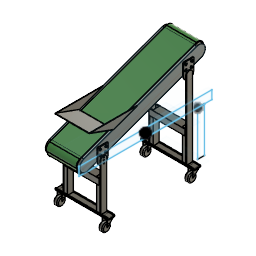
Conveyor Belt with Hopper (Autodesk Fusion 360 design; units mm, degrees)
Autodesk Fusion 360 part; units mm, degrees
note: some values were not read from the file. Chosen so that the rebuilt part matches the saved one: which bodies a step acts on; which face or edge a step refers to. Set by a fixed rule: which sketch regions a step uses.
sketch "Sketch1" plane through (0, 0, 0) normal (1, 0, 0) x (0, 1, 0)
  line L0 (775, 50) -> (-775, 50)
  line L1 (-775, 50) -> (-775, -50)
  line L2 (-775, -50) -> (775, -50)
  line L3 (775, -50) -> (775, 50)
  dimension "d1" = 1550
  dimension "d2" = 100
  constraint horizontal L0
  constraint perpendicular L0 L1
  constraint parallel L0 L2
  constraint parallel L1 L3
  measures "d1" distance of L1.end L2.end
  measures "d2" distance of L0.end L1.end
extrude "Extrude1" add sketch "Sketch1" against normal blind 400 makes body 1
extrude "Extrude2" add 1 faces at (-133.3333, 258.3333, 50) along direction (0, 0, 1) blind 100 on bodies 1 bodies 1
extrude "Extrude3" cut 1 faces at (-133.3333, 258.3333, 150) along direction (0, 0, -1) blind 50 on bodies 1 bodies 1
fillet "Fillet1" radius 75 4 edges at (-200, -775, 100) (-200, -775, -50) (-200, 775, 100) (-200, 775, -50) on bodies 1
sketch "Sketch2" plane through (0, 0, 0) normal (0, 1, 0) x (1, 0, 0)
sketch "Sketch3" plane through (0, 0, 0) normal (1, 0, 0) x (0, 1, 0)
  arc A0 (700, -50) -> (700, 100) centre (700, 25) ccw
  line L0 (700, 100) -> (-700, 100)
  arc A1 (-700, 100) -> (-700, -50) centre (-700, 25) ccw
  line L1 (-700, -50) -> (700, -50)
  line L2 (608.0223, -50) -> (688.0223, -50)
  line L3 (688.0223, -50) -> (688.0223, -570)
  line L4 (688.0223, -570) -> (608.0223, -570)
  line L5 (608.0223, -570) -> (608.0223, -50)
  dimension "d11" = 80
  dimension "d12" = 520
  constraint horizontal L2
  constraint vertical L3
  constraint horizontal L4
  constraint vertical L5
  constraint coincident L1 L2.start
  measures "d11" distance of L2.start L2.end
  measures "d12" distance of L2.start L4.end
sketch "Sketch4" plane through (0, 0, 0) normal (1, 0, 0) x (0, 1, 0)
  arc A0 (700, -50) -> (700, 100) centre (700, 25) ccw
  line L0 (700, 100) -> (-700, 100)
  arc A1 (-700, 100) -> (-700, -50) centre (-700, 25) ccw
  line L1 (-700, -50) -> (700, -50)
  line L2 (655, 125) -> (555, 125)
  line L3 (555, 125) -> (555, -75)
  line L4 (555, -75) -> (655, -75)
  line L5 (655, -75) -> (655, 125)
  point P0 (605, 25)
  dimension "d16" = 100
  dimension "d17" = 200
  constraint horizontal L2
  constraint perpendicular L2 L3
  constraint parallel L2 L4
  constraint parallel L3 L5
  measures "d16" distance of L3.end L4.end
  measures "d17" distance of L2.end L3.end
extrude "Extrude5" add sketch "Sketch4" along normal blind 10 separate body contours L1 L3 L4 L5 | L0 L1 L3 L5 | L0 L2 L3 L5 makes body 2
move_body "Move1" bodies 2 to x (1, 0, 0) y (0, 1, 0) z (0, 0, 1) at (0, 0, -50)
extrude "Extrude6" add 3 faces at (3.3333, 555, 66.6667) (6.6667, 555, 0) (3.3333, 555, -108.3333) along direction (0, -1, 0) blind 20 on bodies 2 bodies 1 2
sketch "Sketch5" plane through (10, 0, 0) normal (1, 0, 0) x (0, 1, 0)
  line L0 (655, -125) -> (655, 75)
  line L1 (655, 75) -> (535, 75)
  line L2 (535, 75) -> (535, -125)
  line L3 (535, -125) -> (655, -125)
  line L4 (595, 75) -> (595, -45)
  line L5 (620, 215) -> (570, 215)
  line L6 (570, 215) -> (570, -305)
  line L7 (570, -305) -> (620, -305)
  line L8 (620, -305) -> (620, 215)
  point P0 (595, -45)
  dimension "d22" = 120
  dimension "d23" = 50
  dimension "d24" = 520
  constraint midpoint L1 L4.start
  constraint perpendicular L1 L4
  constraint horizontal L5
  constraint perpendicular L5 L6
  constraint parallel L5 L7
  constraint parallel L6 L8
  constraint coincident P0 L4.end
  measures "d22" distance of L4.start P0
  measures "d23" distance of L6.end L7.end
  measures "d24" distance of L5.end L6.end
extrude "Extrude7" add sketch "Sketch5" along normal blind 10 separate body contours L3 L6 L7 L8 | L1 L3 L6 L8 | L1 L5 L6 L8 makes body 3
move_body "Move2" bodies 3 to x (1, 0, 0) y (0, 1, 0) z (0, 0, 1) at (0, 0, -260)
move_body "Move3" bodies 3 to x (1, 0, 0) y (0, 1, 0) z (0, 0, 1) at (0, 0, 20)
extrude "Extrude8" add 3 faces at (16.6667, 620, -485) (16.6667, 620, -298.3333) (16.6667, 620, -118.3333) along direction (0, 1, 0) blind 20 on bodies 3 bodies 3
move_body "Move4" bodies 3 to x (1, 0, 0) y (0, 1, 0) z (0, 0, 1) at (0, -10, 0)
fillet "Fillet2" radius 35 2 edges at (15, 630, -25) (15, 560, -25) on bodies 3
fillet "Fillet3" radius 60 2 edges at (5, 535, -125) (5, 655, -125) on bodies 1
sketch "Sketch6" plane through (10, 0, 0) normal (-1, 0, 0) x (0, -1, 0)
  arc A0 (-560, -60) -> (-630, -60) centre (-595, -60) ccw
  line L0 (-630, -60) -> (-630, -545)
  line L1 (-630, -545) -> (-560, -545)
  line L2 (-560, -545) -> (-560, -60)
sketch "Sketch7" plane through (20, 0, 0) normal (1, 0, 0) x (0, 1, 0)
  arc A0 (630, -60) -> (560, -60) centre (595, -60) ccw
  line L0 (560, -60) -> (560, -545)
  line L1 (560, -545) -> (630, -545)
  line L2 (630, -545) -> (630, -60)
  line L3 (595, -25) -> (595, -225)
  line L4 (630, -545) -> (560, -545)
  line L5 (560, -545) -> (560, -225)
  line L6 (560, -225) -> (630, -225)
  line L7 (630, -225) -> (630, -545)
  dimension "d33" = 200
  constraint midpoint A0 L3.start
  constraint vertical L3
  constraint horizontal L4
  constraint vertical L5
  constraint horizontal L6
  constraint vertical L7
  constraint coincident L0 L5.end
  constraint coincident L1.end L2.start
  measures "d33" distance of L3.start L3.end
extrude "Extrude9" add sketch "Sketch7" along normal blind 20 separate body contours L0 L1 L2 L4 L5 L6 L7 makes body 4
move_body "Move5" bodies 4 to x (1, 0, 0) y (0, 1, 0) z (0, 0, 1) at (-30, 0, 0)
extrude "Extrude10" add 1 faces at (-10, 595, -438.3333) along direction (-1, 0, 0) blind 20 on bodies 4 bodies 4
sketch "Sketch8" plane through (0, 0, 0) normal (0, 1, 0) x (1, 0, 0)
sketch "Sketch9" plane through (0, 0, 0) normal (0, 1, 0) x (1, 0, 0)
  line L0 (-50, 190) -> (-450, 190)
  line L1 (-450, 190) -> (-450, 240)
  line L2 (-450, 240) -> (-50, 240)
  line L3 (-50, 240) -> (-50, 190)
  dimension "d38" = 400
  dimension "d39" = 50
  constraint horizontal L0
  constraint vertical L1
  constraint horizontal L2
  constraint vertical L3
  measures "d38" distance of L0.start L0.end
  measures "d39" distance of L0.start L2.end
extrude "Extrude11" add sketch "Sketch9" along normal blind 90 separate body makes body 5
move_body "Move6" bodies 5 to x (1, 0, 0) y (0, 1, 0) z (0, 0, 1) at (50, 550, 30)
extrude "Extrude12" add 1 faces at (-133.3333, 580, -160) along direction (0, 0, 1) blind 20 on bodies 5 bodies 5
sketch "Sketch10" plane through (0, 0, -210) normal (0, 0, -1) x (1, 0, 0)
  line L0 (0, -550) -> (-400, -550)
  line L1 (-400, -550) -> (-400, -640)
  line L2 (-400, -640) -> (0, -640)
  line L3 (0, -640) -> (0, -550)
sketch "Sketch11" plane through (0, 0, -210) normal (0, 0, -1) x (1, 0, 0)
  line L0 (0, -630) -> (-40, -630)
  line L1 (-40, -630) -> (-40, -560)
  line L2 (-40, -560) -> (0, -560)
  line L3 (0, -560) -> (0, -630)
  dimension "d44" = 40
  dimension "d45" = 70
  constraint horizontal L0
  constraint vertical L1
  constraint horizontal L2
  constraint vertical L3
  measures "d44" distance of L0.start L0.end
  measures "d45" distance of L0.start L2.end
sketch "Sketch12" plane through (0, 0, -210) normal (0, 0, -1) x (1, 0, 0)
  line L0 (-400, -630) -> (-360, -630)
  line L1 (-360, -630) -> (-360, -560)
  line L2 (-360, -560) -> (-400, -560)
  line L3 (-400, -560) -> (-400, -630)
  dimension "d46" = 40
  dimension "d47" = 70
  constraint horizontal L0
  constraint vertical L1
  constraint horizontal L2
  constraint vertical L3
  measures "d46" distance of L0.start L0.end
  measures "d47" distance of L0.start L2.end
extrude "Extrude13" cut sketch "Sketch11" sketch "Sketch12" against normal blind 75 of sketch 2 bodies 5
move_body "Move7" bodies 5 to x (1, 0, 0) y (0, 1, 0) z (0, 0, 1) at (10, 0, -40)
sketch "Sketch13" plane through (0, 0, -50) normal (0, 0, -1) x (1, 0, 0)
  line L0 (-400, -700) -> (0, -700)
  line L1 (0, -700) -> (0, -655)
  line L2 (0, -655) -> (0, -535)
  line L3 (0, -535) -> (0, 700)
  line L4 (0, 700) -> (-400, 700)
  line L5 (-400, 700) -> (-400, -700)
sketch "Sketch14" plane through (0, 0, -545) normal (0, 0, -1) x (1, 0, 0)
  line L0 (-30, -630) -> (10, -630)
  line L1 (10, -630) -> (10, -560)
  line L2 (10, -560) -> (-30, -560)
  line L3 (-30, -560) -> (-30, -630)
  line L4 (10, -560) -> (-390, -560)
  line L5 (-390, -560) -> (-390, -610)
  line L6 (-390, -610) -> (10, -610)
  line L7 (10, -610) -> (10, -560)
  dimension "d50" = 400
  dimension "d51" = 50
  constraint horizontal L4
  constraint vertical L5
  constraint horizontal L6
  constraint vertical L7
  constraint coincident L1.end L2.start
  measures "d50" distance of L1.end L4.end
  measures "d51" distance of L1.end L6.end
extrude "Extrude14" add sketch "Sketch14" along normal blind 10 separate body contours L3 L4 L5 L6 | L1 L2 L3 L4 L6 L7 makes body 6
extrude "Extrude15" add 1 faces at (10, 593.3333, -548.3333) along direction (1, 0, 0) blind 100 on bodies 6 bodies 6
extrude "Extrude16" add 1 faces at (-223.3333, 610, -548.3333) along direction (0, 1, 0) blind 20 on bodies 6 bodies 6
extrude "Extrude17" add 1 faces at (-223.3333, 630, -548.3333) along direction (0, 1, 0) blind 5 on bodies 6 bodies 6
sketch "Sketch15" plane through (0, 0, -545) normal (0, 0, 1) x (-1, 0, 0)
  line L0 (390, -635) -> (390, -560)
  line L1 (390, -560) -> (-110, -560)
  line L2 (-110, -560) -> (-110, -635)
  line L3 (-110, -635) -> (390, -635)
sketch "Sketch16" plane through (0, 0, -545) normal (0, 0, 1) x (-1, 0, 0)
  line L0 (-110, -560) -> (390, -560)
  line L1 (390, -560) -> (390, -565)
  line L2 (390, -565) -> (-110, -565)
  line L3 (-110, -565) -> (-110, -560)
  line L4 (-110, -635) -> (390, -635)
  line L5 (390, -635) -> (390, -630)
  line L6 (390, -630) -> (-110, -630)
  line L7 (-110, -630) -> (-110, -635)
  dimension "d60" = 500
  dimension "d61" = 5
  dimension "d62" = 500
  dimension "d63" = 5
  constraint horizontal L0
  constraint vertical L1
  constraint horizontal L2
  constraint vertical L3
  constraint horizontal L4
  constraint vertical L5
  constraint horizontal L6
  constraint vertical L7
  measures "d60" distance of L0.start L0.end
  measures "d61" distance of L0.start L2.end
  measures "d62" distance of L4.start L4.end
  measures "d63" distance of L4.start L6.end
extrude "Extrude18" add sketch "Sketch16" along normal blind 10 bodies 6
sketch "Sketch17" plane through (20, 0, 0) normal (1, 0, 0) x (0, 1, 0)
  arc A0 (630, -60) -> (560, -60) centre (595, -60) ccw
  line L0 (560, -60) -> (560, -545)
  line L1 (560, -545) -> (630, -545)
  line L2 (630, -545) -> (630, -60)
  circle A1 centre (600, -675) radius 50
  dimension "d66" = 100
  measures "d66" diameter of A1
extrude "Extrude19" add sketch "Sketch17" along normal blind 50 separate body contours A1 makes body 7
sketch "Sketch18" plane through (70, 0, 0) normal (1, 0, 0) x (0, 1, 0)
  circle A0 centre (600, -675) radius 50
  line L0 (675, -600) -> (600, -600)
  line L1 (600, -600) -> (600, -675)
  line L2 (600, -675) -> (675, -600)
  dimension "d70" = 75
  constraint horizontal L0
  constraint vertical L1
  constraint coincident A0.centre L1.end
  measures "d70" distance of A0.centre L0.end
extrude "Extrude20" add sketch "Sketch18" along normal blind 5 separate body contours A0 L1 L2 | A0 L0 L1 L2 picked at (618.4794, -647.3437) makes body 8
extrude "Extrude21" add 1 faces at (73.3333, 650, -600) along direction (0, 0, 1) blind 10 on bodies 8 bodies 8
copy_body "CopyPasteBodies1" bodies 8 makes body 9
move_body "Move8" bodies 9 to x (1, 0, 0) y (0, 1, 0) z (0, 0, 1) at (-55, 0, 0)
move_body "Move9" bodies 7 8 9 to x (1, 0, 0) y (0, 1, 0) z (0, 0, 1) at (20, -40, 35)
sketch "Sketch19" plane through (0, 0, 0) normal (1, 0, 0) x (0, 1, 0)
sketch "Sketch20" plane through (0, 0, 0) normal (1, 0, 0) x (0, 1, 0)
  line L0 (-50, 100) -> (-1500, 100)
  line L1 (-1550, 50) -> (-1550, 0)
  line L2 (-1500, -50) -> (-75, -50)
  line L3 (0, 25) -> (0, 50)
  arc A0 (-1550, 0) -> (-1500, -50) centre (-1500, 0) ccw
  arc A1 (-1500, 100) -> (-1550, 50) centre (-1500, 50) ccw
  arc A2 (0, 50) -> (-50, 100) centre (-50, 50) ccw
  arc A3 (-75, -50) -> (0, 25) centre (-75, 25) ccw
  line L4 (-1560, 50) -> (-1560, 0)
  arc A4 (-1560, 0) -> (-1500, -60) centre (-1500, 0) ccw
  line L5 (-1500, -60) -> (-75, -60)
  arc A5 (-75, -60) -> (10, 25) centre (-75, 25) ccw
  line L6 (10, 25) -> (10, 50)
  arc A6 (10, 50) -> (-50, 110) centre (-50, 50) ccw
  line L7 (-50, 110) -> (-1500, 110)
  arc A7 (-1500, 110) -> (-1560, 50) centre (-1500, 50) ccw
  point P0 (-1550, 100)
  point P1 (-1550, -50)
  point P2 (0, -50)
  point P3 (-775, 25)
  dimension "d75" = 1550
  dimension "d76" = 150
  dimension "d77" = 50
  dimension "d78" = 75
  dimension "d79" = 10
  constraint horizontal L0
  constraint perpendicular L0 L1
  constraint parallel L0 L2
  constraint parallel L1 L3
  constraint coincident P1 L2
  constraint coincident P1 L1
  constraint tangent L2 A0
  constraint tangent L1 A0
  constraint coincident P0 L0
  constraint coincident P0 L1
  constraint tangent L0 A1
  constraint tangent L1 A1
  constraint equal A0 A1
  constraint tangent L3 A2
  constraint tangent L0 A2
  constraint equal A0 A2
  constraint coincident P2 L2
  constraint coincident P2 L3
  constraint tangent L2 A3
  constraint tangent L3 A3
  measures "d75" distance of P1 P2
  measures "d76" distance of P0 P1
  measures "d77" radius of A0
  measures "d78" radius of A3
extrude "Extrude22" add sketch "Sketch20" along normal blind 350 separate body makes body 10
move_body "Move10" bodies 10 to x (1, 0, 0) y (0, 1, 0) z (0, 0, 1) at (-375, 780, 0)
sketch "Sketch21" plane through (10, 0, 0) normal (1, 0, 0) x (0, 1, 0)
  arc A0 (535, -65) -> (655, -65) centre (595, -65) ccw
  line L0 (655, -65) -> (655, 75)
  line L1 (655, 75) -> (535, 75)
  line L2 (535, 75) -> (535, -65)
  circle A1 centre (580, 180) radius 12.5
  dimension "d83" = 25
  measures "d83" diameter of A1
extrude "Extrude23" add sketch "Sketch21" along normal blind 5 separate body contours A1 makes body 11
move_body "Move11" bodies 11 to x (1, 0, 0) y (0, 1, 0) z (0, 0, 1) at (0, -20, -130)
move_body "Move12" bodies 11 to x (1, 0, 0) y (0, 1, 0) z (0, 0, 1) at (0, 0, 150)
sketch "Sketch22" plane through (15, 0, 0) normal (1, 0, 0) x (0, 1, 0)
  circle A0 centre (560, 200) radius 12.5
  line L0 (555.3812, 208) -> (550.7624, 200)
  line L1 (550.7624, 200) -> (555.3812, 192)
  line L2 (555.3812, 192) -> (564.6188, 192)
  line L3 (564.6188, 192) -> (569.2376, 200)
  line L4 (569.2376, 200) -> (564.6188, 208)
  line L5 (564.6188, 208) -> (555.3812, 208)
  point P0 (560, 200)
  dimension "d86" = 8
  constraint coincident P0 A0.centre
  measures "d86" distance of P0 L5
extrude "Extrude24" cut sketch "Sketch22" against normal blind 4 contours L0 L1 L2 L3 L4 L5 bodies 11
move_body "Move13" bodies 11 to x (1, 0, 0) y (0, 1, 0) z (0, 0, 1) at (0, 0, -150)
copy_body "CopyPasteBodies2" bodies 11 makes body 12
move_body "Move14" bodies 12 to x (1, 0, 0) y (0, 1, 0) z (0, 0, 1) at (0, 65, 0)
copy_body "CopyPasteBodies3" bodies 11 12 makes body 13 makes body 14
move_body "Move15" bodies 13 14 to x (1, 0, 0) y (0, 1, 0) z (0, 0, 1) at (0, 0, -60)
move_body "Move16" bodies 12 to x (1, 0, 0) y (0, 1, 0) z (0, 0, 1) at (0, 4, 0)
sketch "Sketch23" plane through (10, 0, 0) normal (-1, 0, 0) x (0, -1, 0)
sketch "Sketch24" plane through (20, 0, 0) normal (1, 0, 0) x (0, 1, 0)
  arc A0 (630, -60) -> (560, -60) centre (595, -60) ccw
  line L0 (560, -60) -> (560, -545)
  line L1 (560, -545) -> (630, -545)
  line L2 (630, -545) -> (630, -60)
  circle A1 centre (480, -120) radius 5
  dimension "d89" = 10
  measures "d89" diameter of A1
extrude "Extrude25" add sketch "Sketch24" along normal blind 5 separate body contours A1 makes body 15
sketch "Sketch25" plane through (25, 0, 0) normal (1, 0, 0) x (0, 1, 0)
  circle A0 centre (480, -120) radius 5
  line L0 (477.9793, -116.5) -> (475.9585, -120)
  line L1 (475.9585, -120) -> (477.9793, -123.5)
  line L2 (477.9793, -123.5) -> (482.0207, -123.5)
  line L3 (482.0207, -123.5) -> (484.0415, -120)
  line L4 (484.0415, -120) -> (482.0207, -116.5)
  line L5 (482.0207, -116.5) -> (477.9793, -116.5)
  point P0 (480, -120)
  dimension "d92" = 3.5
  constraint coincident P0 A0.centre
  measures "d92" distance of P0 L5
extrude "Extrude26" cut sketch "Sketch25" against normal blind 4 contours L0 L1 L2 L3 L4 L5 bodies 15
move_body "Move17" bodies 15 to x (1, 0, 0) y (0, 1, 0) z (0, 0, 1) at (0, 115, 80)
move_body "Move18" bodies 15 to x (1, 0, 0) y (0, 1, 0) z (0, 0, 1) at (0, -2, 0)
copy_body "CopyPasteBodies4" bodies 15 makes body 16
move_body "Move19" bodies 16 to x (1, 0, 0) y (0, 1, 0) z (0, 0, 1) at (0, 0, -20)
copy_body "CopyPasteBodies5" bodies 15 makes body 17
move_body "Move20" bodies 17 to x (1, 0, 0) y (0, 1, 0) z (0, 0, 1) at (0, 0, -40)
move_body "Move21" bodies 16 to x (1, 0, 0) y (0, 1, 0) z (0, 0, 1) at (0, 0, -10)
move_body "Move22" bodies 17 to x (1, 0, 0) y (0, 1, 0) z (0, 0, 1) at (0, 0, -20)
sketch "Sketch26" plane through (20, 0, 0) normal (1, 0, 0) x (0, 1, 0)
  arc A0 (630, -60) -> (560, -60) centre (595, -60) ccw
  line L0 (560, -60) -> (560, -545)
  line L1 (560, -545) -> (630, -545)
  line L2 (630, -545) -> (630, -60)
  line L3 (742.0156, -320.3349) -> (703.7134, -288.1956)
  line L4 (697.2855, -295.856) -> (735.5877, -327.9954)
  arc A1 (703.7134, -288.1956) -> (696.6692, -288.8119) centre (700.4994, -292.0258) ccw
  arc A2 (696.6692, -288.8119) -> (697.2855, -295.856) centre (700.4994, -292.0258) ccw
  arc A3 (742.6319, -327.3791) -> (742.0156, -320.3349) centre (738.8017, -324.1652) ccw
  arc A4 (735.5877, -327.9954) -> (742.6319, -327.3791) centre (738.8017, -324.1652) ccw
  point P0 (692.2227, -278.5538)
  point P1 (685.7948, -286.2142)
  point P2 (731.7575, -324.7815)
  point P3 (727.2189, -297.3016)
  dimension "d95" = 60
  dimension "d96" = 10
  dimension "d97" = 5
  constraint parallel L3 L4
  constraint coincident P0 L3
  constraint tangent L3 A1
  constraint coincident P1 L4
  constraint tangent L4 A2
  constraint equal A1 A2
  constraint coincident A1.end A2.start
  constraint tangent L3 A3
  constraint equal A1 A3
  constraint coincident P2 L4
  constraint tangent L4 A4
  constraint equal A1 A4
  constraint coincident A3.start A4.end
  measures "d95" distance of P1 P2
  measures "d96" distance of P0 P1
  measures "d97" radius of A1
extrude "Extrude27" add sketch "Sketch26" along normal blind 1 separate body contours L3 L4 A1 A2 A3 A4 makes body 18
copy_body "CopyPasteBodies6" bodies 18 makes body 19
move_body "Move23" bodies 19 to x (1, 0, 0) y (0, 1, 0) z (0, 0, 1) at (0, 0, -50)
copy_body "CopyPasteBodies7" bodies 18 makes body 20
move_body "Move24" bodies 20 to x (1, 0, 0) y (0, 1, 0) z (0, 0, 1) at (0, 0, -100)
copy_body "CopyPasteBodies8" bodies 18 makes body 21
move_body "Move25" bodies 21 to x (1, 0, 0) y (0, 1, 0) z (0, 0, 1) at (0, 0, -150)
move_body "Move26" bodies 21 20 19 18 to x (1, 0, 0) y (0, 1, 0) z (0, 0, 1) at (0, -125, 100)
move_body "Move27" bodies 19 to x (1, 0, 0) y (0, 1, 0) z (0, 0, 1) at (0, 0, -50)
move_body "Move28" bodies 20 to x (1, 0, 0) y (0, 1, 0) z (0, 0, 1) at (0, 0, -50)
move_body "Move29" bodies 20 to x (1, 0, 0) y (0, 1, 0) z (0, 0, 1) at (0, 0, -50)
move_body "Move30" bodies 21 to x (1, 0, 0) y (0, 1, 0) z (0, 0, 1) at (0, 0, -150)
extrude "Extrude28" cut 4 faces at (21, 589.3381, -201.4622) (21, 589.3381, -301.4622) (21, 589.3381, -401.4622) (21, 589.3381, -501.4622) along direction (-1, 0, 0) blind 10 on bodies 18 19 20 21 bodies 3 18 19 20 21
sketch "Sketch27" plane through (0, 0, 0) normal (1, 0, 0) x (0, 1, 0)
  line L0 (655, -50) -> (685, -50)
  line L1 (685, -50) -> (685, 100)
  line L2 (685, 100) -> (655, 100)
  line L3 (655, 100) -> (655, -50)
  dimension "d102" = 30
  dimension "d103" = 150
  constraint horizontal L0
  constraint vertical L1
  constraint horizontal L2
  constraint vertical L3
  measures "d102" distance of L0.start L0.end
  measures "d103" distance of L0.start L2.end
extrude "Extrude29" add sketch "Sketch27" along normal blind 10 bodies 18 19 20 21
move_body "Move31" bodies 18 to x (1, 0, 0) y (0, 1, 0) z (0, 0, 1) at (10, 0, 0)
move_body "Move32" bodies 18 to x (1, 0, 0) y (0, 1, 0) z (0, 0, 1) at (-10, 0, 0)
extrude "Extrude30" cut 1 faces at (6.6667, 685, 0) along direction (0, -1, 0) blind 10 on bodies 18 bodies 18
sketch "Sketch28" plane through (0, 0, 0) normal (1, 0, 0) x (0, 1, 0)
fillet "Fillet4" radius 10 2 edges at (90, 513.3836, -658.0808) (40, 513.3836, -658.0808) on bodies 7
split "Split1" by plane through (0, 0, 0) normal (1, 0, 0) bodies 1 makes body 22 at (10, 615, -18.3413)
copy_body "CopyPasteBodies9" bodies 22 makes body 23
move_body "Move33" bodies 23 to x (1, 0, 0) y (0, 1, 0) z (0, 0, 1) at (-410, 0, 0)
copy_body "CopyPasteBodies11" bodies 11 makes body 24
move_body "Move34" bodies 24 to x (-1, 0, 0) y (0, 1, 0) z (0, 0, -1) at (-400, 0, 100)
copy_body "CopyPasteBodies12" bodies 24 makes body 25
move_body "Move35" bodies 25 to x (1, 0, 0) y (0, 1, 0) z (0, 0, 1) at (0, 70, 0)
copy_body "CopyPasteBodies13" bodies 24 25 makes body 26 makes body 27
move_body "Move36" bodies 26 27 to x (1, 0, 0) y (0, 1, 0) z (0, 0, 1) at (0, 0, -70)
copy_body "CopyPasteBodies14" bodies 3 makes body 28
move_body "Move37" bodies 28 to x (-1, 0, 0) y (0, -1, 0) z (0, 0, 1) at (-400, 1190, 0)
move_body "Move38" bodies 26 27 to x (1, 0, 0) y (0, 1, 0) z (0, 0, 1) at (0, 0, 10)
copy_body "CopyPasteBodies15" bodies 4 makes body 29
move_body "Move39" bodies 29 to x (1, 0, 0) y (0, 1, 0) z (0, 0, 1) at (-380, 0, 0)
extrude "Extrude31" add 3 faces at (-390, 586.6667, -551.6667) (-390, 561.6667, -541.6667) (-390, 633.3333, -538.3333) along direction (-1, 0, 0) blind 100 on bodies 6 bodies 6
extrude "Extrude32" add 2 faces at (-90, 560, -551.6667) (-90, 560, -538.3333) along direction (0, -1, 0) blind 5 on bodies 6 bodies 6 8 9
extrude "Extrude33" cut 1 faces at (-290, 565, -538.3333) along direction (0, -1, 0) blind 5 on bodies 6 bodies 6
extrude "Extrude34" add 3 faces at (-490, 583.3333, -551.6667) (-490, 633.3333, -538.3333) (-490, 558.3333, -538.3333) along direction (-1, 0, 0) blind 20 on bodies 6 bodies 6
extrude "Extrude35" add 2 faces at (-390, 633.3333, -203.3333) (-390, 553.3333, -203.3333) along direction (-1, 0, 0) blind 20 on bodies 5 bodies 5 28 29
extrude "Extrude36" add 1 faces at (-350, 606.6667, -226.6667) along direction (-1, 0, 0) blind 20 on bodies 5 bodies 5
split "Split2" by plane through (-390, 630, -555) normal (0, 0, -1) bodies 6 makes body 30 at (40, 585, -586.6667) makes body 31 at (95, 585, -586.6667)
copy_body "CopyPasteBodies16" bodies 31 30 makes body 32 makes body 33
move_body "Move40" bodies 32 33 to x (1, 0, 0) y (0, 1, 0) z (0, 0, 1) at (-525, 0, 0)
copy_body "CopyPasteBodies17" bodies 7 makes body 34
move_body "Move41" bodies 34 to x (1, 0, 0) y (0, 1, 0) z (0, 0, 1) at (-525, 0, 0)
copy_body "CopyPasteBodies18" bodies 15 16 17 makes body 35 makes body 36 makes body 37
move_body "Move42" bodies 35 36 37 to x (-1, 0, 0) y (0, -1, 0) z (0, 0, 1) at (-400, 1188, 0)
copy_body "CopyPasteBodies19" bodies 18 makes body 38
move_body "Move43" bodies 38 to x (1, 0, 0) y (0, 1, 0) z (0, 0, 1) at (-410, 0, 0)
copy_body "CopyPasteBodies20" bodies 3 14 5 7 10 6 11 4 13 12 15 16 17 18 22 23 24 25 27 31 34 26 30 38 37 35 36 33 32 makes body 39 makes body 40 makes body 41 makes body 42 makes body 43 makes body 44 makes body 45 makes body 46 makes body 47 makes body 48 makes body 49 makes body 50 makes body 51 makes body 52 makes body 53 makes body 54 makes body 55 makes body 56 makes body 57 makes body 58 makes body 59 makes body 60 makes body 61 makes body 62 makes body 63 makes body 64 makes body 65 makes body 66 makes body 67
move_body "Move44" bodies 39 40 41 42 43 44 45 46 47 48 49 50 51 52 53 54 55 56 57 58 59 60 61 62 63 64 65 66 67 to x (1, 0, 0) y (0, 1, 0) z (0, 0, 1) at (0, -1700, 0)
move_body "Move45" bodies 39 64 62 63 59 58 56 61 60 57 66 67 65 41 45 42 44 46 40 47 52 48 51 55 54 53 50 49 to x (1, 0, 0) y (0, 1, 0) z (0, 0, 1) at (0, 500, 0)
extrude "Extrude37" cut 1 faces at (-375, -1453.3333, 103.3333) along direction (1, 0, 0) blind 700 on bodies 43 bodies 43
move_body "Move46" bodies 52 to x (1, 0, 0) y (0, 1, 0) z (0, 0, 1) at (0, -140, 0)
move_body "Move47" bodies 62 to x (1, 0, 0) y (0, 1, 0) z (0, 0, 1) at (0, -140, 0)
move_body "Move48" bodies 1 to x (1, 0, 0) y (0, 0.766044, 0.642788) z (0, -0.642788, 0.766044) at (0, -213.4549, 486.4626)
move_body "Move49" bodies 10 to x (1, 0, 0) y (0, 0.766044, 0.642788) z (0, -0.642788, 0.766044) at (0, -221.0526, 487.337)
move_body "Move50" bodies 1 to x (1, 0, 0) y (0, 0.984808, -0.173648) z (0, 0.173648, 0.984808) at (0, -9.415, -146.2895)
move_body "Move51" bodies 10 to x (1, 0, 0) y (0, 0.984808, -0.173648) z (0, 0.173648, 0.984808) at (0, -6.9781, -150.7001)
delete_body "RemoveBody1" bodies 52
move_body "Move52" bodies 1 to x (1, 0, 0) y (0, 1, 0) z (0, 0, 1) at (0, 50, 0)
move_body "Move53" bodies 10 to x (1, 0, 0) y (0, 1, 0) z (0, 0, 1) at (0, 50, 0)
move_body "Move54" bodies 1 to x (1, 0, 0) y (0, 0.984808, -0.173648) z (0, 0.173648, 0.984808) at (0, -6.0155, -135.7586)
move_body "Move55" bodies 10 to x (1, 0, 0) y (0, 0.984808, -0.173648) z (0, 0.173648, 0.984808) at (0, -3.0364, -139.4687)
delete_body "RemoveBody2" bodies 62
move_body "Move56" bodies 41 53 61 55 63 50 57 51 59 60 45 40 54 48 65 42 47 46 56 66 39 67 58 49 64 44 to x (1, 0, 0) y (0, 1, 0) z (0, 0, 1) at (0, 50, 0)
delete_body "RemoveBody3" bodies 18
delete_body "RemoveBody4" bodies 38
move_body "Move57" bodies 3 4 37 17 7 13 23 33 25 26 35 27 12 30 22 11 24 34 15 36 14 31 6 5 16 32 to x (1, 0, 0) y (0, 1, 0) z (0, 0, 1) at (0, -50, 0)
move_body "Move58" bodies 40 41 51 50 64 42 67 46 57 49 58 65 56 48 45 59 61 44 47 53 39 63 54 66 55 60 to x (1, 0, 0) y (0, 1, 0) z (0, 0, 1) at (0, 50, 0)
move_body "Move59" bodies 33 7 6 5 4 26 13 17 31 16 35 14 23 24 37 15 11 25 22 36 3 30 12 27 32 34 to x (1, 0, 0) y (0, 1, 0) z (0, 0, 1) at (0, -50, 0)
delete_body "RemoveBody5" bodies 39
split "Split3" by plane through (-410, -520, -545) normal (1, 0, 0) bodies 41 makes body 68 at (-256.6667, -516.6667, -250)
delete_body "RemoveBody6" bodies 41
move_body "Move60" bodies 53 51 50 49 to x (1, 0, 0) y (0, 1, 0) z (0, 0, 1) at (0, 0, 60)
move_body "Move61" bodies 45 48 47 40 to x (1, 0, 0) y (0, 1, 0) z (0, 0, 1) at (0, 0, 60)
move_body "Move62" bodies 54 60 55 56 57 64 65 63 to x (1, 0, 0) y (0, 1, 0) z (0, 0, 1) at (0, 0, 60)
sketch "Sketch29" plane through (0, -115.3844, 317.016) normal (0, -0.34202, 0.939693) x (1, 0, 0)
  line L0 (0, 759.0942) -> (-400, 759.0942)
  line L1 (-400, 759.0942) -> (-400, -640.9058)
  line L2 (-400, -640.9058) -> (0, -640.9058)
  line L3 (0, -640.9058) -> (0, 759.0942)
sketch "Sketch30" plane through (10, 0, 0) normal (1, 0, 0) x (0, 1, 0)
  line L0 (-470, -225) -> (-540, -225)
  line L1 (-540, -225) -> (-540, -545)
  line L2 (-540, -545) -> (-470, -545)
  line L3 (-470, -545) -> (-470, -225)
  line L4 (-540, -545) -> (-470, -545)
  line L5 (-470, -545) -> (-470, -535)
  line L6 (-470, -535) -> (-540, -535)
  line L7 (-540, -535) -> (-540, -545)
  dimension "d124" = 70
  dimension "d125" = 10
  constraint horizontal L4
  constraint vertical L5
  constraint horizontal L6
  constraint vertical L7
  constraint coincident L1.end L2.start
  measures "d124" distance of L1.end L2.end
  measures "d125" distance of L1.end L6.end
extrude "Extrude38" add sketch "Sketch30" along normal blind 10 contours L1 L2 L3 L4 L5 L6 L7 bodies 43 68 46
split "Split4" by plane through (10, -1100, 0) normal (1, 0, 0) bodies 43 makes body 69 at (13.3333, -516.6667, -545)
extrude "Extrude39" add 1 faces at (13.3333, -493.3333, -535) along direction (0, 0, 1) blind 570 on bodies 69 bodies 43 69 49 50 51 53 68
fillet "Fillet5" radius 35 2 edges at (15, -470, 35) (15, -540, 35) on bodies 43
split "Split5" by plane through (10, -470, -535) normal (-1, 0, 0) bodies 43 makes body 70 at (0, -485, 41.6587) makes body 71 at (-256.6667, -516.6667, -250)
copy_body "CopyPasteBodies21" bodies 43 makes body 72
move_body "Move63" bodies 72 to x (1, 0, 0) y (0, 1, 0) z (0, 0, 1) at (-430, 0, 0)
delete_body "RemoveBody7" bodies 3
split "Split6" by plane through (-410, 480, -545) normal (1, 0, 0) bodies 5 makes body 73 at (-256.6667, 483.3333, -250)
delete_body "RemoveBody8" bodies 5
move_body "Move64" bodies 22 17 16 15 13 14 12 11 23 37 36 35 26 24 25 27 to x (1, 0, 0) y (0, 1, 0) z (0, 0, 1) at (0, 0, 420)
copy_body "CopyPasteBodies22" bodies 43 makes body 74
move_body "Move65" bodies 74 to x (1, 0, 0) y (0, 1, 0) z (0, 0, 1) at (0, 1000, 200)
split "Split7" by plane through (20, 1000, 200) normal (1, 0, 0) bodies 74 makes body 75 at (23.3333, 494.3542, 224.8131) makes body 76 at (23.3333, 494.3542, 194.8131) makes body 77 at (23.3333, 494.3542, 164.8131)
delete_body "RemoveBody9" bodies 75
delete_body "RemoveBody10" bodies 76
delete_body "RemoveBody11" bodies 77
move_body "Move66" bodies 74 to x (1, 0, 0) y (0, 1, 0) z (0, 0, 1) at (0, 0, 160)
extrude "Extrude40" add 1 faces at (13.3333, 483.3333, -185) along direction (0, 0, -1) blind 360 on bodies 74 bodies 4 74 73
split "Split8" by plane through (10, 530, -175) normal (-1, 0, 0) bodies 4 makes body 78 at (-256.6667, 483.3333, -250)
copy_body "CopyPasteBodies23" bodies 43 makes body 79
copy_body "CopyPasteBodies24" bodies 4 makes body 80
move_body "Move67" bodies 80 to x (1, 0, 0) y (0, 1, 0) z (0, 0, 1) at (-430, 0, 0)
sketch "Sketch31" plane through (0, 0, 0) normal (1, 0, 0) x (0, 1, 0)
  line L0 (-666.3358, -43.1406) -> (649.2338, 435.6876)
  arc A0 (649.2338, 435.6876) -> (597.9308, 576.6415) centre (623.5823, 506.1645) ccw
  line L1 (597.9308, 576.6415) -> (-717.6389, 97.8133)
  arc A1 (-717.6389, 97.8133) -> (-666.3358, -43.1406) centre (-691.9873, 27.3363) ccw
sketch "Sketch32" plane through (0, 0, 0) normal (1, 0, 0) x (0, 1, 0)
sketch "Sketch33" plane through (0, 0, 0) normal (1, 0, 0) x (0, 1, 0)
  line L0 (-379.7645, 414.6018) -> (-97.8567, 517.2079)
  line L1 (-379.7645, 414.6018) -> (-79.7645, 414.6018) construction
  line L2 (-379.7645, 414.6018) -> (-379.7645, 517.2079)
  line L3 (-379.7645, 517.2079) -> (-97.8567, 517.2079)
  line L4 (-97.8567, 517.2079) -> (-661.6723, 517.2079)
  line L5 (-661.6723, 517.2079) -> (-379.7645, 414.6018)
  dimension "d134" = 300
  dimension "d135" = 20
  dimension "d136" = 102.606
  dimension "d137" = 281.9078
  dimension "d138" = 563.8156
  constraint horizontal L1
  constraint vertical L2
  constraint perpendicular L2 L3
  constraint parallel L3 L4
  measures "d134" distance of L0.start L0.end
  measures "d135" angle of L0 L1
  measures "d136" distance of L0.start L2.end
  measures "d137" distance of L2.end L0.end
  measures "d138" distance of L0.end L4.end
extrude "Extrude41" add sketch "Sketch33" along normal blind 5 separate body makes body 81
copy_body "CopyPasteBodies25" bodies 81 makes body 82
move_body "Move68" bodies 82 to x (1, 0, 0) y (0, 1, 0) z (0, 0, 1) at (-400, 0, 0)
sketch "Sketch34" plane through (0, 88.8264, 244.0487) normal (0, -0.34202, -0.939693) x (1, 0, 0)
  line L0 (-400, 798.6641) -> (-400, 498.6641)
  line L1 (-400, 498.6641) -> (-395, 498.6641)
  line L2 (-395, 498.6641) -> (-395, 798.6641)
  line L3 (-395, 798.6641) -> (-400, 798.6641)
  line L4 (-395, 798.6641) -> (0, 798.6641)
  line L5 (0, 798.6641) -> (0, 498.66)
  line L6 (0, 498.66) -> (-395, 498.66)
  line L7 (-395, 498.66) -> (-395, 798.6641)
  constraint horizontal L4
  constraint vertical L5
  constraint horizontal L6
  constraint vertical L7
  constraint coincident L2.end L3.start
extrude "Extrude42" add sketch "Sketch34" against normal blind 5 contours L2 L4 L5 L6 L7 bodies 81 82
move_body "Move69" bodies 81 to x (1, 0, 0) y (0, 1, 0) z (0, 0, 1) at (0, 0, -200)
move_body "Move70" bodies 81 to x (1, 0, 0) y (0, 1, 0) z (0, 0, 1) at (0, 0, 10)
equation "d138 = ( 2 * 281.9077862 ) * 1 mm"
